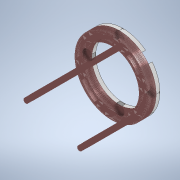
# Autodesk Inventor part: Top holder magnet
Saved by Autodesk Inventor 2022.4 (Build 264492010, 492A)
## iProperties
Created: 2023-01-04
Part Number: Top holder magnet
Material: Generic
Document SubType Name: Modeling
Designer: tmass
Density: 1 g/cm^3
Appearance: Default
Author: tmass
Autodesk Inventor part; units mm, degrees
ref_plane "YZ Plane" through (0, 0, 0) normal (1, 0, 0) x (0, 1, 0)
ref_plane "XZ Plane" through (0, 0, 0) normal (0, 1, 0) x (-1, 0, 0)
sketch "Sketch1" plane through (15.1716, 31.1499, -10) normal (0, 0, -1) x (-1, 0, 0)
  circle A0 centre (15.1718, 2.3509) radius 5.5
  circle A1 centre (15.1682, -31.1568) radius 39.0078 projected
  line L0 (15.1682, 16.6184) -> (15.1682, -92.5886) construction
  line L1 (67.6065, -31.1568) -> (-2.4603, -31.1568) construction
  circle A2 centre (-18.3396, -31.1532) radius 5.5
  circle A3 centre (15.1646, -64.6646) radius 5.5
  circle A4 centre (48.676, -31.1605) radius 5.5
  circle A5 centre (15.1721, -31.1497) radius 28.9995 projected
  circle A6 centre (15.1721, -31.1497) radius 39.0149
  circle A7 centre (15.1721, -31.1497) radius 28.9995
  point P0 (15.1716, -31.1499)
  point P1 (-17.7938, -52.0162)
  point P2 (15.182, -70.1646)
  point P3 (-13.6795, -34.0745)
  point P4 (-13.6801, -28.231)
  point P5 (18.083, -60.0028)
  point P6 (12.2483, -60.0015)
  point P7 (54.176, -31.1611)
  point P8 (54.176, -31.1568)
  dimension "d0" = 11
  dimension "d3" = 360
  constraints: 6 centre point, 4 end point, 2 coincident, 1 concentric, 1 horizontal, 1 tangent, 1 vertical, 9 other
  measures "d0" diameter of A0
extrude "Extrusion1" add sketch "Sketch1" along normal blind 4 contours A0 A5 | A0 A1 A4 A5 | A1 A6 | A0 A5 A2 A1 | A1 A4 A5 | A2 A5 A3 A1 | A2 A5 | A1 A3 A5 A4 | A3 A5 picked at (15.172, 1.1724) picked at (-17.1539, -31.1527) picked at (15.165, -63.4768)
extrude "Extrusion2" cut sketch "Sketch1" along normal blind 3.5 contours A0 A5 | A0 A5 | A1 A4 A5 | A2 A5 | A5 A4 | A3 A5 picked at (-17.1539, -31.1527) picked at (15.165, -63.4768)
sketch "Sketch3" plane through (0, 0, 0) normal (0, 1, 0) x (-1, 0, 0)
  point P0 (0, 0)
sketch "Sketch4" plane through (15.1716, 31.1499, -14) normal (0, 0, -1) x (-1, 0, 0)
  line L0 (15.1716, -11.9634) -> (15.1716, -53.9026)
  line L1 (30.3972, -46.3755) -> (6.4991, -22.4774)
  point P0 (15.1716, -31.1499)
  dimension "d9" = 135
  constraints: 4 end point, 2 point on line, 1 vertical
  measures "d9" angle of L0 L1
ref_plane "Work Plane1" through (-15.2256, -15.2256, -14) normal (0.7071, -0.7071, 0) x (0.7071, 0.7071, 0)
sketch "Sketch5" plane through (-15.2256, -15.2256, -14) normal (0.7071, -0.7071, 0) x (0.7071, 0.7071, 0)
  line L0 (50.5315, 0) -> (50.5315, 4) projected
  line L1 (50.5315, -1.9282) -> (46.5682, 5.2134)
  line L2 (46.5682, 5.2134) -> (63.3976, 5.2134)
  line L3 (63.3976, 5.2134) -> (68.7285, -4.3924)
  line L4 (68.7285, -4.3924) -> (51.8991, -4.3924)
  line L5 (51.8991, -4.3924) -> (50.5315, -1.9282)
  point P0 (21.5323, 14)
  constraints: 10 end point, 2 parallel, 2 point on line, 1 collinear, 1 perpendicular
extrude "Extrusion3" cut sketch "Sketch5" along normal mid plane 10
body "Solid1"
